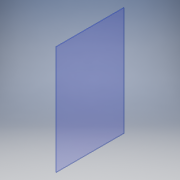
# Autodesk Inventor part: BellyPan
Saved by Autodesk Inventor 2019 (Build 230136000, 136)
## iProperties
Created: 2020-01-24
Part Number: BellyPan
Material: Generic
Document SubType Name: Modeling
Designer: james
Density: 1 g/cm^3
Appearance: Clear - Blue
Author: james
Autodesk Inventor part; units mm, degrees
ref_plane "YZ Plane" through (0, 0, 0) normal (1, 0, 0) x (0, 1, 0)
ref_plane "XZ Plane" through (0, 0, 0) normal (0, 1, 0) x (-1, 0, 0)
ref_plane "XY Plane" through (0, 0, 0) normal (0, 0, 1) x (1, 0, 0)
sketch "Sketch1" plane through (0, 0, 0) normal (1, 0, 0) x (0, 1, 0)
  line L0 (796.0794, 324.8073) -> (-10.3706, 324.8073)
  line L1 (-10.3706, 324.8073) -> (-10.3706, -176.8427)
  line L2 (-10.3706, -176.8427) -> (796.0794, -176.8427)
  line L3 (796.0794, -176.8427) -> (796.0794, 324.8073)
  point P0 (0, 0)
  dimension "d0" = 501.65
  dimension "d1" = 806.45
  constraints: 8 end point, 2 parallel, 1 horizontal, 1 perpendicular
  measures "d0" distance of L0.end L1.end
  measures "d1" distance of L0.start L0.end
extrude "Extrusion1" add sketch "Sketch1" along normal blind 4.7625
body "Solid1"
